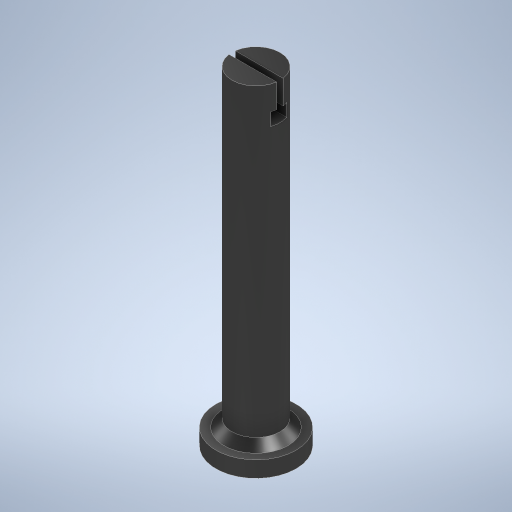
# Autodesk Inventor part: Taster
Saved by Autodesk Inventor 2023.1 (Build 271208000, 208)
## iProperties
Created: 2023-12-10
Part Number: Taster
Material: Generic
Document SubType Name: Modeling
Designer: JansenL
Density: 1 g/cm^3
Appearance: Glossy - Black
Author: JansenL
Autodesk Inventor part; units mm, degrees
ref_plane "YZ Plane" through (0, 0, 0) normal (1, 0, 0) x (0, 1, 0)
ref_plane "XZ Plane" through (0, 0, 0) normal (0, 1, 0) x (-1, 0, 0)
ref_plane "XY Plane" through (0, 0, 0) normal (0, 0, 1) x (1, 0, 0)
sketch "Sketch1" plane through (0, 0, 0) normal (0, 0, 1) x (1, 0, 0)
  line L0 (0, 0) -> (0, 26)
  line L1 (0, 26) -> (1.5, 26)
  line L2 (1.5, 26) -> (1.5, 1)
  line L3 (1.5, 1) -> (2.5, 1)
  line L4 (2.5, 1) -> (2.5, 0)
  line L5 (2.5, 0) -> (0, 0)
  line L6 (1.5, 26) -> (4, 26)
  line L7 (4, 26) -> (4, 24)
  line L8 (4, 24) -> (1.5, 24)
  line L9 (1.5, 24) -> (1.5, 26)
  point P0 (1.5, 24)
  dimension "d0" = 2.5
  dimension "d1" = 1.5
  dimension "d2" = 1
  dimension "d3" = 26
  dimension "d5" = 2
  dimension "d6" = 4
  constraints: 20 end point, 6 perpendicular, 2 parallel, 1 horizontal, 1 vertical
  measures "d0" distance between parallel lines of L0 L4
  measures "d1" distance of L0.end L1.end
  measures "d2" distance between parallel lines of L5 L3
  measures "d3" distance between parallel lines of L5 L1
  measures "d5" distance between parallel lines of L8 L6
  measures "d6" distance between parallel lines of L7 L0
revolve "Revolution1" add sketch "Sketch1" angle 360 about axis through (0, 0, 0) along (0, 1, 0) contours L0 L1 L2 L3 L4 L5
sketch "Sketch2" plane through (0, 0, 0) normal (0, -1, 0) x (1, 0, 0)
  circle A0 centre (0, 0) radius 1.6
  dimension "d10" = 3.2
  constraints: 1 centre point, 1 coincident
  measures "d10" diameter of A0
extrude "Extrusion1" cut sketch "Sketch2" against normal blind 0.5
chamfer "Chamfer1" distance 0.5 angle 45 1 edges at (-1.5, 1, 0)
sketch "Sketch3" plane through (0, 0, 0) normal (1, 0, 0) x (0, 1, 0)
  line L0 (1.5, 1.5) -> (26, 1.5) projected
  line L1 (20.5, 1.5) -> (20.5, 0.2)
  line L2 (20.5, 0.2) -> (19, 0.2)
  line L3 (19, 0.2) -> (19, 0.5)
  line L4 (19, 0.5) -> (18.2, 0.5)
  line L5 (18.2, 0.5) -> (18.2, -0.5)
  line L6 (18.2, -0.5) -> (19, -0.5)
  line L7 (19, -0.5) -> (19, -0.2)
  line L8 (19, -0.2) -> (20.5, -0.2)
  line L9 (20.5, -0.2) -> (20.5, -1.5)
  line L10 (1.5, -1.5) -> (26, -1.5) projected
  line L11 (26, 0) -> (62.914, 0) construction
  line L12 (20.5, 1.5) -> (26, 1.5)
  line L13 (1.5, 1.5) -> (26, 1.5) projected
  line L14 (26, -1.5) -> (26, 1.5) projected
  line L15 (26, -1.5) -> (26, 1.5)
  line L16 (26, 1.5) -> (26, -1.5)
  line L17 (20.5, -1.5) -> (26, -1.5)
  line L18 (26, 0) -> (18.2, 0) construction
  point P0 (0, 0)
  dimension "d16" = 0.4
  dimension "d17" = 1.5
  dimension "d18" = 0.8
  dimension "d19" = 1
  dimension "d23" = 5.5
  dimension "d24" = 1.3
  constraints: 30 end point, 9 perpendicular, 5 collinear, 2 point on line, 1 horizontal, 1 midpoint, 1 vertical, 2 other
  measures "d16" distance between parallel lines of L8 L2
  measures "d17" distance between parallel lines of L3 L1
  measures "d18" distance of L3.end L4.end
  measures "d19" distance of L4.end L5.end
  measures "d23" distance between parallel lines of L1 L15
  measures "d24" distance between parallel lines of L0 L2
extrude "Extrusion2" cut sketch "Sketch3" along normal mid plane 10
body "Solid1"
